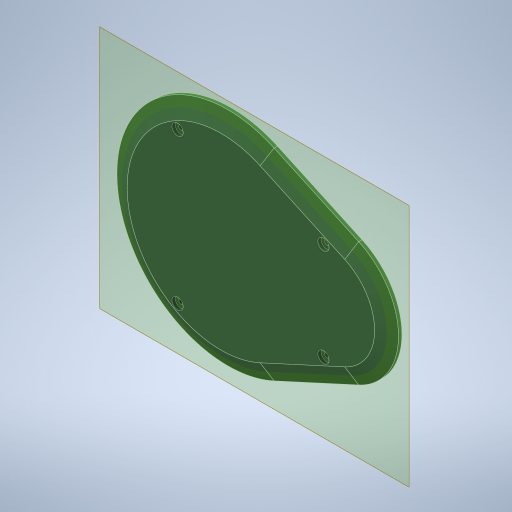
# Autodesk Inventor part: Wirst_2R_cover
Saved by Autodesk Inventor 2023 (Build 270158000, 158)
## iProperties
Created: 2024-07-25
Part Number: Wirst_2R_cover
Material: Generic
Document SubType Name: Modeling
Designer: Swoby
Density: 1 g/cm^3
Appearance: Default
Author: Swoby
Autodesk Inventor part; units mm, degrees
ref_plane "YZ Plane" through (0, 0, 0) normal (1, 0, 0) x (0, 1, 0)
ref_plane "XZ Plane" through (0, 0, 0) normal (0, 1, 0) x (-1, 0, 0)
ref_plane "XY Plane" through (0, 0, 0) normal (0, 0, 1) x (1, 0, 0)
sketch "Sketch1" plane through (0, 0, 0) normal (0, 0, 1) x (1, 0, 0)
  arc A0 (13.5417, 29.5444) -> (13.5417, -29.5444) centre (0, 0) ccw
  arc A1 (38.3333, -18.1812) -> (38.3333, 18.1812) centre (30, 0) ccw
  line L0 (0, 0) -> (30, 0)
  line L1 (13.5417, 29.5444) -> (38.3333, 18.1812)
  line L2 (13.5417, -29.5444) -> (38.3333, -18.1812)
  dimension "d0" = 65
  dimension "d1" = 40
  dimension "d2" = 30
  constraints: 6 end point, 4 point on circle, 4 tangent, 2 centre point, 1 coincident, 1 horizontal
  measures "d0" diameter of A0
  measures "d1" diameter of A1
  measures "d2" distance of point (0, 0) L0.end
extrude "Extrusion1" add sketch "Sketch1" along normal blind 3
chamfer "Chamfer1" distance 5 distance2 2 4 edges at (50, 0, 3) (25.9375, 23.8628, 3) (-32.5, 0, 3) (25.9375, -23.8628, 3) measured on face at (-32, 0, 3) measured on face at (25.7292, 23.4083, 3) measured on face at (25.7292, -23.4083, 3) measured on face at (49.5, 0, 3)
sketch "Sketch2" plane through (0, 0, 0) normal (0, 0, -1) x (-1, 0, 0)
  line L0 (-13.5417, -29.5444) -> (-38.3333, -18.1812) construction
  arc A0 (-13.5417, -29.5444) -> (-13.5417, 29.5444) centre (0, 0) ccw construction
  line L1 (-38.3333, 18.1812) -> (-13.5417, 29.5444) construction
  arc A1 (-38.3333, 18.1812) -> (-38.3333, -18.1812) centre (-30, 0) ccw construction
  arc A2 (-10.625, -23.181) -> (-10.625, 23.181) centre (0, 0) ccw construction
  line L2 (-10.625, -23.181) -> (-35.4167, -11.8178) construction
  arc A3 (-35.4167, 11.8178) -> (-35.4167, -11.8178) centre (-30, 0) ccw construction
  line L3 (-35.4167, 11.8178) -> (-10.625, 23.181) construction
  line L4 (0, 0) -> (12.75, 22.0836) construction
  line L5 (0, 0) -> (12.75, -22.0836) construction
  line L6 (-30, 14.3005) -> (-30, -14.3005) construction
  circle A4 centre (-30, 14.3005) radius 0.65
  circle A5 centre (-30, -14.3005) radius 0.65
  circle A6 centre (12.75, -22.0836) radius 0.65
  circle A7 centre (12.75, 22.0836) radius 0.65
  dimension "d8" = 7
  dimension "d9" = 30
  dimension "d10" = 30
  dimension "d11" = 1.3
  dimension "d12" = 1.3
  dimension "d13" = 1.3
  dimension "d14" = 1.3
  constraints: 10 end point, 6 centre point, 6 point on circle, 4 coincident, 2 point on line, 1 midpoint, 1 vertical, 3 other
  measures "d8" distance between parallel lines of L1 L3
  measures "d9" angle of L6 L4
  measures "d10" angle of L6 L5
  measures "d11" diameter of A4
  measures "d12" diameter of A5
  measures "d13" diameter of A6
  measures "d14" diameter of A7
extrude "Extrusion2" cut sketch "Sketch2" against normal blind 10
ref_plane "Work Plane1" through (0, 0, 2) normal (0, 0, -1) x (-1, 0, 0)
sketch "Sketch3" plane through (0, 0, 2) normal (0, 0, -1) x (-1, 0, 0)
  circle A0 centre (12.75, -22.0836) radius 0.65 projected
  circle A1 centre (-30, -14.3005) radius 0.65 projected
  circle A2 centre (12.75, 22.0836) radius 0.65 projected
  circle A3 centre (-30, 14.3005) radius 0.65 projected
  line L0 (-13.5417, -29.5444) -> (-38.3333, -18.1812) projected
  arc A4 (-13.5417, -29.5444) -> (-13.5417, 29.5444) centre (0, 0) ccw projected
  line L1 (-38.3333, 18.1812) -> (-13.5417, 29.5444) projected
  arc A5 (-38.3333, 18.1812) -> (-38.3333, -18.1812) centre (-30, 0) ccw projected
  circle A6 centre (-30, 14.3005) radius 1.65
  circle A7 centre (-30, -14.3005) radius 1.65
  circle A8 centre (12.75, -22.0836) radius 1.65
  circle A9 centre (12.75, 22.0836) radius 1.65
  dimension "d18" = 3.3
  dimension "d19" = 3.3
  dimension "d20" = 3.3
  dimension "d21" = 3.3
  constraints: 4 centre point, 4 coincident
  measures "d18" diameter of A6
  measures "d19" diameter of A7
  measures "d20" diameter of A8
  measures "d21" diameter of A9
extrude "Extrusion3" cut sketch "Sketch3" against normal blind 10 contours A0 | A1 | A2 | A3 | A6 | A7 | A8 | A9
body "Solid1"
